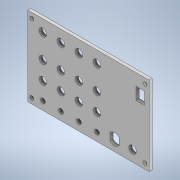
# Autodesk Inventor part: Box Top
Saved by Autodesk Inventor 2022 (Build 260153000, 153)
## iProperties
Created: 2021-07-04
Part Number: Box Top
Material: Generic
Document SubType Name: Modeling
Designer: Matthijs
Density: 1 g/cm^3
Appearance: Default
Author: Matthijs
Autodesk Inventor part; units mm, degrees
ref_plane "YZ Plane" through (0, 0, 0) normal (1, 0, 0) x (0, 1, 0)
ref_plane "XZ Plane" through (0, 0, 0) normal (0, 1, 0) x (-1, 0, 0)
ref_plane "XY Plane" through (0, 0, 0) normal (0, 0, 1) x (1, 0, 0)
sketch "Sketch1" plane through (0, 0, 0) normal (0, 0, 1) x (1, 0, 0)
  line L0 (100.775, -66.125) -> (-100.775, -66.125)
  line L1 (-100.775, -66.125) -> (-100.775, 66.125)
  line L2 (-100.775, 66.125) -> (100.775, 66.125)
  line L3 (100.775, 66.125) -> (100.775, -66.125)
  line L4 (100.775, -66.125) -> (-100.775, 66.125) construction
  line L5 (-100.775, -66.125) -> (100.775, 66.125) construction
  point P0 (0, 0)
  dimension "d0" = 201.55
  dimension "d1" = 132.25
  constraints: 12 end point, 2 midpoint, 2 parallel, 1 horizontal, 1 perpendicular
  measures "d0" distance of L1.end L2.end
  measures "d1" distance of L0.end L1.end
extrude "TopPlate" add sketch "Sketch1" along normal blind 5
sketch "Sketch2" plane through (0, 0, 5) normal (0, 0, 1) x (1, 0, 0)
  line L0 (-100.775, -66.125) -> (100.775, -66.125) projected
  line L1 (-100.775, -66.125) -> (-87.775, -66.125)
  line L2 (-87.775, -66.125) -> (-87.775, -48.125)
  line L3 (-87.775, -48.125) -> (-100.775, -48.125)
  line L4 (-100.775, -48.125) -> (-100.775, -66.125)
  line L5 (100.775, -66.125) -> (100.775, 66.125) projected
  line L6 (100.775, -66.125) -> (87.775, -66.125)
  line L7 (87.775, -66.125) -> (87.775, -48.125)
  line L8 (87.775, -48.125) -> (100.775, -48.125)
  line L9 (100.775, -48.125) -> (100.775, -66.125)
  line L10 (100.775, 66.125) -> (-100.775, 66.125) projected
  line L11 (-100.775, 66.125) -> (-87.775, 66.125)
  line L12 (-87.775, 66.125) -> (-87.775, 48.125)
  line L13 (-87.775, 48.125) -> (-100.775, 48.125)
  line L14 (-100.775, 48.125) -> (-100.775, 66.125)
  line L15 (100.775, 66.125) -> (87.775, 66.125)
  line L16 (87.775, 66.125) -> (87.775, 48.125)
  line L17 (87.775, 48.125) -> (100.775, 48.125)
  line L18 (100.775, 48.125) -> (100.775, 66.125)
  line L19 (-100.775, 66.125) -> (-87.775, 48.125)
  line L20 (-87.775, 66.125) -> (-100.775, 48.125)
  line L21 (87.775, 66.125) -> (100.775, 48.125)
  line L22 (100.775, 48.125) -> (100.775, 66.125)
  line L23 (87.775, 48.125) -> (100.775, 66.125)
  line L24 (100.775, -66.125) -> (87.775, -48.125)
  line L25 (100.775, -48.125) -> (87.775, -66.125)
  line L26 (-100.775, -48.125) -> (-87.775, -66.125)
  line L27 (-100.775, 66.125) -> (-100.775, -66.125) projected
  line L28 (-87.775, -48.125) -> (-100.775, -66.125)
  point P0 (0, 0)
  point P1 (-94.275, -57.125)
  point P2 (-94.275, 57.125)
  point P3 (94.275, 57.125)
  point P4 (94.275, -57.125)
  dimension "d4" = 13
  dimension "d5" = 18
  dimension "d6" = 13
  dimension "d7" = 18
  dimension "d8" = 13
  dimension "d9" = 18
  dimension "d10" = 13
  dimension "d11" = 18
  constraints: 50 end point, 9 parallel, 4 horizontal, 4 midpoint, 4 perpendicular, 2 point on line, 1 vertical
  measures "d4" distance of L3.end L2.end
  measures "d5" distance of L2.end L1.end
  measures "d6" distance of L7.end L8.end
  measures "d7" distance of L6.end L7.end
  measures "d8" distance of L12.end L13.end
  measures "d9" distance of L11.end L12.end
  measures "d10" distance of L17.end L16.end
  measures "d11" distance of L16.end L15.end
hole "Hole1" at (-94.275, -57.125, 5) at (94.275, 57.125, 5) at (94.275, -57.125, 5) at (-94.275, 57.125, 5) direction (0, 0, -1) diameter 3.4 end through all counterbore diameter 6.5 counterbore depth 3.4 clearance for "Socket Head Cap Screw DIN EN ISO 4762" size "M3" standard "DIN"
sketch "Sketch34" plane through (0, 0, 5) normal (0, 0, 1) x (1, 0, 0)
  circle A0 centre (73.525, -47.875) radius 6.25
  line L0 (100.775, 66.125) -> (-100.775, 66.125) projected
  line L1 (-100.775, 66.125) -> (-100.775, -66.125) projected
  line L2 (-100.775, -66.125) -> (100.775, -66.125) projected
  point P0 (0, 0)
  point P1 (-125, -13.875)
  point P2 (-125, 66.125)
  point P3 (-125, 66.125)
  point P4 (-65, 66.125)
  dimension "d166" = 12.5
  dimension "d170" = 174.3
  dimension "d261" = 18.25
  constraints: 1 centre point
  measures "d166" diameter of A0
  measures "d170" distance from line of L1 A0.centre
  measures "d261" distance from line of L2 A0.centre
extrude "ToggleswitchWithCap1" cut sketch "Sketch34" against normal blind 10
sketch "Sketch38" plane through (0, 0, 5) normal (0, 0, 1) x (1, 0, 0)
  line L0 (79.225, 46.125) -> (93.225, 46.125)
  line L1 (93.225, 46.125) -> (93.225, 26.125)
  line L2 (93.225, 26.125) -> (79.225, 26.125)
  line L3 (79.225, 26.125) -> (79.225, 46.125)
  line L4 (100.775, 66.125) -> (-100.775, 66.125) projected
  line L5 (-100.775, 66.125) -> (-100.775, -66.125) projected
  point P0 (0, 0)
  dimension "d181" = 14
  dimension "d182" = 20
  dimension "d185" = 20
  dimension "d186" = 180
  constraints: 8 end point, 2 parallel, 1 horizontal, 1 perpendicular
  measures "d181" distance of L1.end L2.end
  measures "d182" distance of L0.end L1.end
  measures "d185" distance between parallel lines of L4 L0
  measures "d186" distance between parallel lines of L5 L3
extrude "OnOffToggle" cut sketch "Sketch38" against normal through all
sketch "Sketch17" plane through (0, 0, 5) normal (0, 0, 1) x (1, 0, 0)
  circle A0 centre (43.525, -47.875) radius 9.5
  line L0 (100.775, 66.125) -> (-100.775, 66.125) projected
  line L1 (-100.775, 66.125) -> (-100.775, -66.125) projected
  line L2 (-100.775, -66.125) -> (100.775, -66.125) projected
  point P0 (0, 0)
  point P1 (-104.4472, 75)
  point P2 (-85.5528, 75)
  point P3 (-125, -57.3222)
  point P4 (-125, -38.4278)
  dimension "d81" = 19
  dimension "d83" = 144.3
  dimension "d223" = 18.25
  constraints: 1 centre point
  measures "d81" diameter of A0
  measures "d83" distance from line of L1 A0.centre
  measures "d223" distance from line of L2 A0.centre
extrude "KeySwitch" cut sketch "Sketch17" against normal through all
sketch "Sketch18" plane through (0, 0, 5) normal (0, 0, 1) x (1, 0, 0)
  circle A0 centre (-75.775, 46.625) radius 6.25
  line L0 (-100.775, 66.125) -> (-100.775, -66.125) projected
  line L1 (100.775, 66.125) -> (-100.775, 66.125) projected
  line L2 (100.775, -66.125) -> (100.775, 66.125) projected
  point P0 (0, 0)
  point P1 (-11.1695, 75)
  point P2 (1.1695, 75)
  dimension "d86" = 12.5
  dimension "d99" = 19.5
  dimension "d225" = 25
  constraints: 1 centre point
  measures "d86" diameter of A0
  measures "d99" distance from line of L1 A0.centre
  measures "d225" distance from line of L0 A0.centre
extrude "Toggleswitch1" cut sketch "Sketch18" against normal through all
sketch "Sketch19" plane through (0, 0, 5) normal (0, 0, 1) x (1, 0, 0)
  circle A0 centre (-45.775, 46.625) radius 6.25
  line L0 (100.775, 66.125) -> (-100.775, 66.125) projected
  line L1 (-100.775, 66.125) -> (-100.775, -66.125) projected
  line L2 (100.775, -66.125) -> (100.775, 66.125) projected
  point P0 (0, 0)
  dimension "d89" = 12.5
  dimension "d100" = 19.5
  dimension "d226" = 55
  constraints: 1 centre point
  measures "d89" diameter of A0
  measures "d100" distance from line of L0 A0.centre
  measures "d226" distance from line of L1 A0.centre
extrude "Toggleswitch2" cut sketch "Sketch19" against normal through all
sketch "Sketch20" plane through (0, 0, 5) normal (0, 0, 1) x (1, 0, 0)
  circle A0 centre (-15.775, 46.625) radius 6.25
  line L0 (100.775, 66.125) -> (-100.775, 66.125) projected
  line L1 (-100.775, 66.125) -> (-100.775, -66.125) projected
  line L2 (100.775, -66.125) -> (100.775, 66.125) projected
  point P0 (0, 0)
  dimension "d92" = 12.5
  dimension "d102" = 19.5
  dimension "d227" = 85
  constraints: 1 centre point
  measures "d92" diameter of A0
  measures "d102" distance from line of L0 A0.centre
  measures "d227" distance from line of L1 A0.centre
extrude "Toggleswitch3" cut sketch "Sketch20" against normal through all
sketch "Sketch21" plane through (0, 0, 5) normal (0, 0, 1) x (1, 0, 0)
  circle A0 centre (14.225, 46.625) radius 6.25
  line L0 (100.775, 66.125) -> (-100.775, 66.125) projected
  line L1 (-100.775, 66.125) -> (-100.775, -66.125) projected
  line L2 (100.775, -66.125) -> (100.775, 66.125) projected
  point P0 (0, 0)
  dimension "d95" = 12.5
  dimension "d104" = 19.5
  dimension "d228" = 115
  constraints: 1 centre point
  measures "d95" diameter of A0
  measures "d104" distance from line of L0 A0.centre
  measures "d228" distance from line of L1 A0.centre
extrude "Toggleswitch4" cut sketch "Sketch21" against normal through all
sketch "Sketch22" plane through (0, 0, 5) normal (0, 0, 1) x (1, 0, 0)
  circle A0 centre (-75.775, 6.625) radius 6.1
  line L0 (-100.775, 66.125) -> (-100.775, -66.125) projected
  line L1 (100.775, 66.125) -> (-100.775, 66.125) projected
  line L2 (100.775, -66.125) -> (100.775, 66.125) projected
  point P0 (0, 0)
  dimension "d106" = 12.2
  dimension "d110" = 59.5
  dimension "d229" = 25
  constraints: 1 centre point
  measures "d106" diameter of A0
  measures "d110" distance from line of L1 A0.centre
  measures "d229" distance from line of L0 A0.centre
extrude "ButtonBlack1" cut sketch "Sketch22" against normal through all
sketch "Sketch23" plane through (0, 0, 5) normal (0, 0, 1) x (1, 0, 0)
  circle A0 centre (-45.775, 6.625) radius 6.1
  line L0 (100.775, 66.125) -> (-100.775, 66.125) projected
  line L1 (-100.775, 66.125) -> (-100.775, -66.125) projected
  line L2 (100.775, -66.125) -> (100.775, 66.125) projected
  point P0 (0, 0)
  dimension "d111" = 12.2
  dimension "d114" = 59.5
  dimension "d230" = 55
  constraints: 1 centre point
  measures "d111" diameter of A0
  measures "d114" distance from line of L0 A0.centre
  measures "d230" distance from line of L1 A0.centre
extrude "ButtonBlack2" cut sketch "Sketch23" against normal through all
sketch "Sketch24" plane through (0, 0, 5) normal (0, 0, 1) x (1, 0, 0)
  circle A0 centre (-15.775, 6.625) radius 6.1
  line L0 (100.775, 66.125) -> (-100.775, 66.125) projected
  line L1 (-100.775, 66.125) -> (-100.775, -66.125) projected
  line L2 (100.775, -66.125) -> (100.775, 66.125) projected
  point P0 (0, 0)
  dimension "d116" = 12.2
  dimension "d117" = 59.5
  dimension "d231" = 85
  constraints: 1 centre point
  measures "d116" diameter of A0
  measures "d117" distance from line of L0 A0.centre
  measures "d231" distance from line of L1 A0.centre
extrude "ButtonBlack3" cut sketch "Sketch24" against normal through all
sketch "Sketch25" plane through (0, 0, 5) normal (0, 0, 1) x (1, 0, 0)
  circle A0 centre (14.225, 6.625) radius 6.1
  line L0 (100.775, 66.125) -> (-100.775, 66.125) projected
  line L1 (-100.775, 66.125) -> (-100.775, -66.125) projected
  line L2 (100.775, -66.125) -> (100.775, 66.125) projected
  point P0 (0, 0)
  dimension "d121" = 12.2
  dimension "d205" = 59.5
  dimension "d232" = 115
  constraints: 1 centre point
  measures "d121" diameter of A0
  measures "d205" distance from line of L0 A0.centre
  measures "d232" distance from line of L1 A0.centre
extrude "ButtonBlack4" cut sketch "Sketch25" against normal through all
sketch "Sketch26" plane through (0, 0, 5) normal (0, 0, 1) x (1, 0, 0)
  circle A0 centre (-75.775, -23.375) radius 6.1
  line L0 (-100.775, 66.125) -> (-100.775, -66.125) projected
  line L1 (100.775, 66.125) -> (-100.775, 66.125) projected
  line L2 (100.775, -66.125) -> (100.775, 66.125) projected
  point P0 (0, 0)
  dimension "d126" = 12.2
  dimension "d128" = 89.5
  dimension "d233" = 25
  constraints: 1 centre point
  measures "d126" diameter of A0
  measures "d128" distance from line of L1 A0.centre
  measures "d233" distance from line of L0 A0.centre
extrude "ButtonRed1" cut sketch "Sketch26" against normal through all
sketch "Sketch27" plane through (0, 0, 5) normal (0, 0, 1) x (1, 0, 0)
  circle A0 centre (-45.775, -23.375) radius 6.1
  line L0 (100.775, 66.125) -> (-100.775, 66.125) projected
  line L1 (-100.775, 66.125) -> (-100.775, -66.125) projected
  line L2 (100.775, -66.125) -> (100.775, 66.125) projected
  point P0 (0, 0)
  dimension "d131" = 12.2
  dimension "d132" = 89.5
  dimension "d234" = 55
  constraints: 1 centre point
  measures "d131" diameter of A0
  measures "d132" distance from line of L0 A0.centre
  measures "d234" distance from line of L1 A0.centre
extrude "ButtonRed2" cut sketch "Sketch27" against normal through all
sketch "Sketch28" plane through (0, 0, 5) normal (0, 0, 1) x (1, 0, 0)
  circle A0 centre (-15.775, -23.375) radius 6.1
  line L0 (100.775, 66.125) -> (-100.775, 66.125) projected
  line L1 (-100.775, 66.125) -> (-100.775, -66.125) projected
  line L2 (100.775, -66.125) -> (100.775, 66.125) projected
  point P0 (0, 0)
  dimension "d136" = 12.2
  dimension "d137" = 89.5
  dimension "d235" = 85
  constraints: 1 centre point
  measures "d136" diameter of A0
  measures "d137" distance from line of L0 A0.centre
  measures "d235" distance from line of L1 A0.centre
extrude "ButtonRed3" cut sketch "Sketch28" against normal through all
sketch "Sketch29" plane through (0, 0, 5) normal (0, 0, 1) x (1, 0, 0)
  circle A0 centre (14.225, -23.375) radius 6.1
  line L0 (100.775, 66.125) -> (-100.775, 66.125) projected
  line L1 (-100.775, 66.125) -> (-100.775, -66.125) projected
  line L2 (100.775, -66.125) -> (100.775, 66.125) projected
  point P0 (0, 0)
  dimension "d141" = 12.2
  dimension "d142" = 89.5
  dimension "d236" = 115
  constraints: 1 centre point
  measures "d141" diameter of A0
  measures "d142" distance from line of L0 A0.centre
  measures "d236" distance from line of L1 A0.centre
extrude "ButtonRed4" cut sketch "Sketch29" against normal through all
sketch "Sketch39" plane through (0, 0, 5) normal (0, 0, 1) x (1, 0, 0)
  line L0 (-85.775, -40.2112) -> (36.025, -40.2112)
  line L1 (36.025, -40.2112) -> (36.025, -66.125)
  line L2 (36.025, -66.125) -> (-85.775, -66.125)
  line L3 (-85.775, -66.125) -> (-85.775, -40.2112)
  circle A0 centre (43.525, -47.875) radius 9.5 projected
  line L4 (-100.775, -66.125) -> (100.775, -66.125) projected
  line L5 (-100.775, 66.125) -> (-100.775, -66.125) projected
  point P0 (0, 0)
  point P1 (36.025, -53.706)
  point P2 (36.025, -42.044)
  dimension "d187" = 7.5
  dimension "d218" = 0
  dimension "d224" = 15
  constraints: 8 end point, 2 parallel, 1 horizontal, 1 perpendicular
  measures "d187" distance from line of A0.centre L1
  measures "d218" distance between parallel lines of L4 L2
  measures "d224" distance between parallel lines of L5 L3
extrude "KeySwitchSideLeft" add sketch "Sketch39" against normal up to surface (5 mm away) contours L0 L1 A0 L2 L3 | L1 A0 picked at (35.6607, -49.2254)
sketch "Sketch40" plane through (0, 0, 5) normal (0, 0, 1) x (1, 0, 0)
  line L0 (51.025, -34.9523) -> (60.7775, -34.9523)
  line L1 (60.7775, -34.9523) -> (60.7775, -58.7516)
  line L2 (60.7775, -58.7516) -> (51.025, -58.7516)
  line L3 (51.025, -58.7516) -> (51.025, -34.9523)
  arc A0 (36.025, -53.706) -> (36.025, -42.044) centre (43.525, -47.875) ccw projected
  point P0 (0, 0)
  point P1 (51.025, -42.044)
  point P2 (51.025, -53.706)
  dimension "d190" = 7.5
  constraints: 8 end point, 2 parallel, 1 horizontal, 1 perpendicular
  measures "d190" distance from line of A0.centre L3
extrude "KeySwitchSideRight" add sketch "Sketch40" against normal up to surface (5 mm away) contours A0 L3
sketch "Sketch44" plane through (0, 0, 5) normal (0, 0, 1) x (1, 0, 0)
  circle A0 centre (-75.775, -52.275) radius 4
  line L0 (-100.775, 66.125) -> (-100.775, -66.125) projected
  line L1 (100.775, 66.125) -> (-100.775, 66.125) projected
  point P0 (0, 0)
  dimension "d241" = 8
  dimension "d253" = 25
  dimension "d254" = 118.4
  constraints: 1 centre point
  measures "d241" diameter of A0
  measures "d253" distance from line of L0 A0.centre
  measures "d254" distance from line of L1 A0.centre
extrude "RotaryEncoder1" cut sketch "Sketch44" against normal through all
sketch "Sketch45" plane through (0, 0, 5) normal (0, 0, 1) x (1, 0, 0)
  circle A0 centre (-45.775, -52.275) radius 4
  line L0 (100.775, 66.125) -> (-100.775, 66.125) projected
  line L1 (-100.775, 66.125) -> (-100.775, -66.125) projected
  point P0 (0, 0)
  dimension "d244" = 8
  dimension "d255" = 118.4
  dimension "d256" = 55
  constraints: 1 centre point
  measures "d244" diameter of A0
  measures "d255" distance from line of L0 A0.centre
  measures "d256" distance from line of L1 A0.centre
extrude "RotaryEncoder2" cut sketch "Sketch45" against normal through all
sketch "Sketch46" plane through (0, 0, 5) normal (0, 0, 1) x (1, 0, 0)
  circle A0 centre (-15.775, -52.275) radius 4
  line L0 (100.775, 66.125) -> (-100.775, 66.125) projected
  line L1 (-100.775, 66.125) -> (-100.775, -66.125) projected
  point P0 (0, 0)
  dimension "d247" = 8
  dimension "d257" = 118.4
  dimension "d258" = 85
  constraints: 1 centre point
  measures "d247" diameter of A0
  measures "d257" distance from line of L0 A0.centre
  measures "d258" distance from line of L1 A0.centre
extrude "RotaryEncoder3" cut sketch "Sketch46" against normal through all
sketch "Sketch47" plane through (0, 0, 5) normal (0, 0, 1) x (1, 0, 0)
  circle A0 centre (14.225, -52.275) radius 4
  line L0 (100.775, 66.125) -> (-100.775, 66.125) projected
  line L1 (-100.775, 66.125) -> (-100.775, -66.125) projected
  point P0 (0, 0)
  dimension "d250" = 8
  dimension "d259" = 118.4
  dimension "d260" = 115
  constraints: 1 centre point
  measures "d250" diameter of A0
  measures "d259" distance from line of L0 A0.centre
  measures "d260" distance from line of L1 A0.centre
extrude "RotaryEncoder4" cut sketch "Sketch47" against normal through all
body "Solid1"
